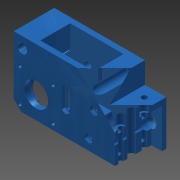
# Autodesk Inventor part: YAxisMotorBlock
Saved by Autodesk Inventor 2015 (Build 190159000, 159)
## iProperties
Created: 2014-08-06
Part Number: YAxisMotorBlock
Material: ABS Plastic
Document SubType Name: Modeling
Designer: t_clevj
Density: 1.06 g/cm^3
Appearance: Cyan
Author: t_clevj
Autodesk Inventor part; units mm, degrees
ref_plane "YZ Plane" through (0, 0, 0) normal (1, 0, 0) x (0, 1, 0)
ref_plane "XZ Plane" through (0, 0, 0) normal (0, 1, 0) x (-1, 0, 0)
ref_plane "XY Plane" through (0, 0, 0) normal (0, 0, 1) x (1, 0, 0)
sketch "Sketch1" plane through (0, 0, 0) normal (0, 1, 0) x (-1, 0, 0)
  line L0 (0, 0) -> (105, 0)
  line L1 (105, 0) -> (105, 62)
  line L2 (105, 62) -> (20, 62)
  line L3 (20, 62) -> (20, 42)
  line L4 (20, 42) -> (0, 42)
  line L5 (0, 42) -> (0, 0)
  dimension "d0" = 105
  dimension "d1" = 62
  dimension "d2" = 85
  dimension "d3" = 20
  constraints: 12 end point, 4 perpendicular, 2 horizontal
  measures "d0" distance of L0.start L0.end
  measures "d1" distance of L0.end L1.end
  measures "d2" distance of L1.end L2.end
  measures "d3" distance of L2.end L3.end
extrude "BottomFace" add sketch "Sketch1" along normal blind 5
sketch "Sketch2" plane through (0, 5, 0) normal (0, 1, 0) x (1, 0, 0)
  line L0 (0, 0) -> (-105, 0) projected
  line L1 (-105, 0) -> (-105, -62) projected
  line L2 (-93, -6.5778) -> (-93, 0)
  line L3 (-105, -62) -> (-20, -62) projected
  line L4 (-85, -62) -> (-85, -37.9706)
  arc A0 (-93, -6.5778) -> (-85, -37.9706) centre (-84, -21) ccw
  line L5 (-20, -42) -> (0, -42) projected
  line L6 (-20, -62) -> (-20, -42) projected
  line L7 (0, -42) -> (0, 0) projected
  arc A1 (-30, -46) -> (-19, -35) centre (-30, -35) ccw
  line L8 (-19, -35) -> (-19, 0)
  line L9 (-35, -46) -> (-35, -62)
  line L10 (-30, -46) -> (-35, -46)
  line L11 (-46, -10) -> (-71.0385, -10)
  line L12 (-73, -8.0385) -> (-73, 0)
  arc A2 (-42.5498, -2) -> (-46, -10) centre (-35, -10) ccw
  line L13 (-42.5498, -2) -> (-42.5498, 0)
  arc A3 (-71.0385, -10) -> (-73, -8.0385) centre (-84, -21) ccw
  dimension "d30" = 34
  dimension "d31" = 21
  dimension "d32" = 21
  dimension "d33" = 20
  dimension "d35" = 12
  dimension "d38" = 22
  dimension "d39" = 27
  dimension "d40" = 30
  dimension "d41" = 15
  dimension "d44" = 20
  dimension "d45" = 22
  dimension "d46" = 10
  dimension "d47" = 35
  dimension "d48" = 2
  dimension "d51" = 17
  dimension "d52" = 10
  constraints: 16 end point, 8 point on circle, 6 perpendicular, 6 point on line, 4 centre point, 2 tangent, 1 coincident, 1 horizontal, 1 vertical
  measures "d30" diameter of A0
  measures "d31" distance from line of L1 A0.centre
  measures "d32" distance from line of L0 A0.centre
  measures "d33" distance between parallel lines of L1 L4
  measures "d35" distance from line of L0.end L2
  measures "d38" diameter of A1
  measures "d39" distance from line of L3 A1.centre
  measures "d40" distance from line of L7 A1.centre
  measures "d41" distance between parallel lines of L6 L9
  measures "d44" distance between parallel lines of L2 L12
  measures "d45" diameter of A2
  measures "d46" distance from line of L0 A2.centre
  measures "d47" distance from line of L7 A2.centre
  measures "d48" distance of L13.start L13.end
  measures "d51" radius of A3
  measures "d52" distance between parallel lines of L0 L11
extrude "Extrusion9" add sketch "Sketch2" along normal blind 28 contours L7 L5 L6 L3 L9 L10 A1 L8 L0 | L13 A2 L11 A3 L12 L0 | L2 A0 L4 L3 L1 L0
sketch "Sketch8" plane through (0, 5, 0) normal (0, 1, 0) x (1, 0, 0)
  arc A0 (-93, -6.5778) -> (-85, -37.9706) centre (-84, -21) ccw projected
  circle A1 centre (-84, -21) radius 11.25
  line L0 (-105, 0) -> (-105, -62) projected
  line L1 (-42.5498, 0) -> (-73, 0) projected
  point P0 (0, 0)
  dimension "d53" = 22.5
  constraints: 1 centre point, 1 coincident
  measures "d53" diameter of A1
extrude "Extrusion10" cut sketch "Sketch8" against normal up to next
sketch "Sketch9" plane through (0, 33, 0) normal (0, 1, 0) x (1, 0, 0)
  line L0 (-20, -42) -> (0, -42) projected
  line L1 (0, -42) -> (0, 0) projected
  line L2 (0, 0) -> (-105, 0) projected
  line L3 (-10, 0) -> (-10, -37)
  line L4 (-10, -37) -> (0, -37)
  dimension "d62" = 5
  dimension "d63" = 10
  constraints: 4 end point, 2 point on line, 1 perpendicular, 1 vertical
  measures "d62" distance between parallel lines of L0 L4
  measures "d63" distance between parallel lines of L1 L3
extrude "Extrusion11" cut sketch "Sketch9" against normal up to next
sketch "Sketch10" plane through (0, 33, 0) normal (0, 1, 0) x (1, 0, 0)
  line L0 (0, -37) -> (-10, -37) projected
  line L1 (-10, -37) -> (-10, 0) projected
  line L2 (-20, -62) -> (-20, -42) projected
  line L3 (-20, -42) -> (0, -42) projected
  line L4 (0, -42) -> (0, -37) projected
  line L5 (-105, 0) -> (-105, -62) projected
  line L6 (-105, -62) -> (-85, -62) projected
  line L7 (-85, -62) -> (-85, -37.9706) projected
  arc A0 (-93, -6.5778) -> (-85, -37.9706) centre (-84, -21) ccw projected
  line L8 (-93, -6.5778) -> (-93, 0) projected
  line L9 (-93, 0) -> (-105, 0) projected
  line L10 (-71.0385, -10) -> (-46, -10) projected
  arc A1 (-42.5498, -2) -> (-46, -10) centre (-35, -10) ccw projected
  line L11 (-42.5498, -2) -> (-42.5498, 0) projected
  line L12 (-42.5498, 0) -> (-73, 0) projected
  line L13 (-73, 0) -> (-73, -8.0385) projected
  arc A2 (-71.0385, -10) -> (-73, -8.0385) centre (-84, -21) ccw projected
  line L14 (-20, -62) -> (-105, -62)
  line L15 (-105, -62) -> (-105, 0)
  line L16 (-105, 0) -> (-10, 0)
  point P0 (0, 0)
  constraints: 6 end point, 1 collinear, 1 horizontal, 1 perpendicular
extrude "Extrusion12" add sketch "Sketch10" along normal blind 5
sketch "Sketch11" plane through (0, 5, 0) normal (0, 1, 0) x (1, 0, 0)
  arc A0 (-30, -46) -> (-19, -35) centre (-30, -35) ccw projected
  arc A1 (-42.5498, -2) -> (-46, -10) centre (-35, -10) ccw projected
  circle A2 centre (-35, -10) radius 2.25
  circle A3 centre (-30, -35) radius 2.25
  point P0 (0, 0)
  dimension "d68" = 4.5
  dimension "d69" = 4.5
  constraints: 2 centre point, 2 coincident
  measures "d68" diameter of A2
  measures "d69" diameter of A3
extrude "Extrusion13" cut sketch "Sketch11" along normal blind 39.5 and the other way blind 5
sketch "Sketch13" plane through (0, 38, 0) normal (0, 1, 0) x (1, 0, 0)
  circle A0 centre (-99.5, -5.5) radius 1.75
  circle A1 centre (-68.5, -5.5) radius 1.75
  circle A2 centre (-68.5, -36.5) radius 1.75
  circle A3 centre (-99.5, -36.5) radius 1.75
  circle A4 centre (-84, -21) radius 11.25 projected
  point P0 (0, 0)
  dimension "d78" = 3.5
  dimension "d79" = 31
  dimension "d80" = 31
  dimension "d81" = 15.5
  dimension "d82" = 15.5
  constraints: 4 centre point, 3 equal radius, 2 horizontal alignment, 2 vertical alignment
  measures "d78" diameter of A0
  measures "d79" distance of A0.centre A1.centre
  measures "d80" distance of A2.centre A1.centre
  measures "d81" horizontal distance of A4.centre A2.centre
  measures "d82" horizontal distance of A4.centre A1.centre
hole "Hole1" at (-68.5, 38, 36.5) at (-68.5, 38, 5.5) at (-99.5, 38, 5.5) at (-99.5, 38, 36.5) direction (0, -1, 0) diameter 3.5 end up to face face through (-68.3369, 0, 51.8396) facing (0, -1, 0) counterbore diameter 6 counterbore depth 34
sketch "Sketch14" plane through (0, 0, 0) normal (0, -1, 0) x (1, 0, 0)
  line L0 (-20, 62) -> (-20, 42) projected
  line L1 (-105, 62) -> (-20, 62) projected
  line L2 (-105, 0) -> (-105, 62) projected
  circle A0 centre (-97, 52) radius 2.5
  circle A1 centre (-28, 52) radius 2.5
  point P0 (0, 0)
  dimension "d90" = 5
  dimension "d91" = 5
  dimension "d92" = 10
  dimension "d93" = 8
  dimension "d94" = 8
  constraints: 2 centre point, 1 horizontal alignment
  measures "d90" diameter of A0
  measures "d91" diameter of A1
  measures "d92" distance from line of L1 A1.centre
  measures "d93" distance from line of L2 A0.centre
  measures "d94" distance from line of L0 A1.centre
hole "Hole2" at (-28, 0, 52) at (-97, 0, 52) direction (0, 1, 0) diameter 5.5 end up to face face through (-64.3795, 38, 54.4927) facing (0, 1, 0) counterbore diameter 9 counterbore depth 33
fillet "Fillet1" radius 5 2 edges at (-35, 19, 46) (-85, 19, 37.9706)
sketch "Sketch15" plane through (0, 38, 0) normal (0, 1, 0) x (1, 0, 0)
  line L0 (-10, 0) -> (-105, 0) projected
  line L1 (-105, 0) -> (-105, -62) projected
  line L2 (-56.5, -38) -> (-56.5, -23) construction
  line L3 (-54.25, -38) -> (-54.25, -23)
  line L4 (-58.75, -23) -> (-58.75, -38)
  arc A0 (-58.75, -38) -> (-54.25, -38) centre (-56.5, -38) ccw
  arc A1 (-54.25, -23) -> (-58.75, -23) centre (-56.5, -23) ccw
  circle A2 centre (-56.5, -38) radius 3.5 construction
  point P0 (0, 0)
  point P1 (-56.5, -30.5)
  dimension "d103" = 7.5
  dimension "d104" = 4.5
  dimension "d105" = 48.5
  dimension "d106" = 23
  dimension "d118" = 7
  constraints: 8 end point, 4 point on circle, 4 tangent, 3 centre point, 1 coincident, 1 midpoint, 1 parallel, 1 vertical
  measures "d103" distance of point (-56.5, -30.5) L2.end
  measures "d104" diameter of A1
  measures "d105" distance between parallel lines of L1 L2
  measures "d106" distance from line of L0 L2.end
  measures "d118" diameter of A2
extrude "Extrusion15" cut sketch "Sketch15" against normal up to surface (38 mm away)
sketch "Sketch16" plane through (0, 0, 0) normal (0, -1, 0) x (1, 0, 0)
  line L0 (-54.25, 38) -> (-54.25, 23) projected
  arc A0 (-58.75, 23) -> (-54.25, 23) centre (-56.5, 23) ccw projected
  line L1 (-58.75, 23) -> (-58.75, 38) projected
  arc A1 (-54.25, 38) -> (-58.75, 38) centre (-56.5, 38) ccw projected
  line L2 (-56.5, 42.0415) -> (-53, 40.0207)
  line L3 (-53, 40.0207) -> (-53, 35.9793)
  line L4 (-53, 35.9793) -> (-56.5, 33.9585)
  line L5 (-56.5, 33.9585) -> (-60, 35.9793)
  line L6 (-60, 35.9793) -> (-60, 40.0207)
  line L7 (-60, 40.0207) -> (-56.5, 42.0415)
  line L8 (-56.5, 18.9585) -> (-60, 20.9793)
  line L9 (-60, 20.9793) -> (-60, 25.0207)
  line L10 (-60, 25.0207) -> (-56.5, 27.0415)
  line L11 (-56.5, 27.0415) -> (-53, 25.0207)
  line L12 (-53, 25.0207) -> (-53, 20.9793)
  line L13 (-53, 20.9793) -> (-56.5, 18.9585)
  line L14 (-60, 35.9793) -> (-60, 25.0207)
  line L15 (-53, 35.9793) -> (-53, 25.0207)
  point P0 (0, 0)
  dimension "d109" = 7
  constraints: 28 end point, 3 vertical, 2 coincident, 1 collinear, 1 vertical alignment, 26 other
  measures "d109" distance between parallel lines of L9 L12
extrude "Extrusion16" cut sketch "Sketch16" against normal blind 3.2
sketch "Sketch17" plane through (0, 0, 0) normal (0, -1, 0) x (1, 0, 0)
  circle A0 centre (-35, 10) radius 2.25 projected
  circle A1 centre (-30, 35) radius 2.25 projected
  line L0 (-35, 5.9585) -> (-38.5, 7.9793)
  line L1 (-38.5, 7.9793) -> (-38.5, 12.0207)
  line L2 (-38.5, 12.0207) -> (-35, 14.0415)
  line L3 (-35, 14.0415) -> (-31.5, 12.0207)
  line L4 (-31.5, 12.0207) -> (-31.5, 7.9793)
  line L5 (-31.5, 7.9793) -> (-35, 5.9585)
  line L6 (-30, 30.9585) -> (-33.5, 32.9793)
  line L7 (-33.5, 32.9793) -> (-33.5, 37.0207)
  line L8 (-33.5, 37.0207) -> (-30, 39.0415)
  line L9 (-30, 39.0415) -> (-26.5, 37.0207)
  line L10 (-26.5, 37.0207) -> (-26.5, 32.9793)
  line L11 (-26.5, 32.9793) -> (-30, 30.9585)
  point P0 (0, 0)
  dimension "d112" = 7
  constraints: 24 end point, 2 coincident, 2 vertical, 1 parallel, 26 other
  measures "d112" distance between parallel lines of L10 L7
extrude "Extrusion17" cut sketch "Sketch17" against normal blind 3.2
sketch "Sketch18" plane through (-10, 0, 0) normal (0, 0, -1) x (-1, 0, 0)
  line L0 (0, 38) -> (0, 0) projected
  circle A0 centre (0, 15.5) radius 4
  line L1 (0, 38) -> (95, 38) projected
  line L2 (0, 38) -> (0, 0) projected
  point P0 (-10, 0)
  dimension "d115" = 8
  dimension "d192" = 22.5
  constraints: 1 centre point, 1 point on line
  measures "d115" diameter of A0
  measures "d192" distance from line of L1 A0.centre
extrude "Extrusion18" cut sketch "Sketch18" against normal up to surface (37 mm away)
sketch "Sketch21" plane through (0, 0, 37) normal (0, 0, -1) x (-1, 0, 0)
  line L0 (0, 38) -> (10, 38) projected
  line L1 (10, 0) -> (0, 0) projected
  line L2 (10, 11.5) -> (10, 0) projected
  circle A0 centre (10, 30) radius 4.25
  circle A1 centre (10, 8) radius 4.25
  line L3 (10, 38) -> (10, 19.5) projected
  dimension "d125" = 8.5
  dimension "d126" = 8.5
  dimension "d127" = 8
  dimension "d128" = 8
  constraints: 2 centre point, 2 point on line
  measures "d125" diameter of A0
  measures "d126" diameter of A1
  measures "d127" distance from line of L0 A0.centre
  measures "d128" distance from line of L1 A1.centre
extrude "Extrusion21" [suppressed]
sketch "Sketch22" plane through (-10, 30, 37) normal (0, 0, -1) x (-1, 0, 0)
  circle A0 centre (0, 0) radius 4.25 projected
  circle A1 centre (0, -22) radius 4.25 projected
  circle A2 centre (0, -22) radius 2.5
  circle A3 centre (0, 0) radius 2.5
  point P0 (-10, -30)
  dimension "d133" = 5
  dimension "d134" = 5
  constraints: 2 centre point, 2 coincident
  measures "d133" diameter of A2
  measures "d134" diameter of A3
extrude "Extrusion22" [suppressed]
sketch "Sketch23" plane through (0, 38, 0) normal (0, 1, 0) x (1, 0, 0)
  line L0 (-54.25, -23) -> (-54.25, -38) projected
  arc A0 (-58.75, -38) -> (-54.25, -38) centre (-56.5, -38) ccw projected
  line L1 (-58.75, -38) -> (-58.75, -23) projected
  arc A1 (-54.25, -23) -> (-58.75, -23) centre (-56.5, -23) ccw projected
  line L2 (-56.5, -38) -> (-56.5, -23) construction
  line L3 (-53, -38) -> (-53, -23)
  line L4 (-60, -23) -> (-60, -38)
  arc A2 (-60, -38) -> (-53, -38) centre (-56.5, -38) ccw
  arc A3 (-53, -23) -> (-60, -23) centre (-56.5, -23) ccw
  point P0 (0, 0)
  point P1 (-56.5, -30.5)
  dimension "d137" = 7
  constraints: 8 end point, 4 point on circle, 4 tangent, 2 centre point, 1 midpoint, 1 parallel, 1 vertical
  measures "d137" diameter of A3
extrude "Extrusion23" cut sketch "Sketch23" against normal blind 4
sketch "Sketch24" plane through (-10, 38, 37) normal (1, 0, 0) x (0, 0, -1)
  line L0 (37, 0) -> (37, -18.5) projected
  line L1 (0, 0) -> (0, -18.5) projected
  line L2 (37, -38) -> (0, -38) projected
  line L3 (37, -26.5) -> (37, -38) projected
  line L4 (37, -26.5) -> (0, -26.5) projected
  circle A0 centre (31, -10.5) radius 2
  circle A1 centre (31, -32.5) radius 2
  line L5 (0, -26.5) -> (0, -38) projected
  line L6 (0, -18.5) -> (37, -18.5) projected
  line L7 (37, 0) -> (37, -18.5) projected
  line L8 (0, 0) -> (37, 0) projected
  dimension "d140" = 4
  dimension "d141" = 4
  dimension "d144" = 6
  dimension "d210" = 5.5
  dimension "d212" = 27.5
  constraints: 2 centre point, 1 vertical alignment
  measures "d140" diameter of A0
  measures "d141" diameter of A1
  measures "d144" distance from line of L0 A0.centre
  measures "d210" distance from line of L2 A1.centre
  measures "d212" distance from line of L2 A0.centre
extrude "Extrusion24" cut sketch "Sketch24" against normal up to surface (9 mm away) contours A0 | A1
sketch "Sketch25" plane through (-10, 38, 37) normal (1, 0, 0) x (0, 0, -1)
  line L0 (37, 0) -> (37, -18.5) projected
  line L1 (0, 0) -> (37, 0) projected
  line L2 (0, 0) -> (0, -18.5) projected
  line L3 (0, -4) -> (37, -4)
  dimension "d147" = 4
  constraints: 2 end point, 2 point on line, 1 perpendicular
  measures "d147" distance between parallel lines of L1 L3
extrude "Extrusion25" add sketch "Sketch25" along normal blind 10
sketch "Sketch26" plane through (-10, 34, 0) normal (0, -1, 0) x (1, 0, 0)
  line L0 (0, 0) -> (10, 0) projected
  line L1 (10, 37) -> (10, 0) projected
  circle A0 centre (0, 18.5) radius 2.5
  dimension "d150" = 5
  dimension "d151" = 10
  dimension "d152" = 18.5
  constraints: 1 centre point
  measures "d150" diameter of A0
  measures "d151" distance from line of L1 A0.centre
  measures "d152" distance from line of L0 A0.centre
extrude "Extrusion26" cut sketch "Sketch26" against normal up to next
sketch "Sketch27" plane through (0, 0, 37) normal (0, 0, -1) x (-1, 0, 0)
  line L0 (0, 0) -> (0, 34) projected
  circle A0 centre (10, 27.5) radius 2.5
  circle A1 centre (10, 5.5) radius 2.5
  line L1 (10, 0) -> (0, 0) projected
  dimension "d155" = 5
  dimension "d156" = 5
  dimension "d157" = 10
  dimension "d207" = 5.5
  dimension "d208" = 27.5
  constraints: 2 centre point, 1 vertical alignment
  measures "d155" diameter of A0
  measures "d156" diameter of A1
  measures "d157" distance from line of L0 A0.centre
  measures "d207" distance from line of L1 A1.centre
  measures "d208" distance from line of L1 A0.centre
extrude "Extrusion27" cut sketch "Sketch27" against normal up to next
sketch "Sketch28" plane through (-10, 0, 0) normal (0, 0, -1) x (-1, 0, 0)
  circle A0 centre (0, 27.5) radius 2.5 projected
  arc A1 (0, 25) -> (0, 30) centre (0, 27.5) ccw projected
  arc A2 (0, 30) -> (0, 25) centre (0, 27.5) ccw projected
  circle A3 centre (0, 5.5) radius 2.5 projected
  arc A4 (0, 3) -> (0, 8) centre (0, 5.5) ccw projected
  arc A5 (0, 8) -> (0, 3) centre (0, 5.5) ccw projected
  point P0 (-10, 0)
extrude "Extrusion28" cut sketch "Sketch28" against normal blind 37
sketch "Sketch29" plane through (0, 0, 37) normal (0, 0, -1) x (-1, 0, 0)
  circle A0 centre (10, 27.5) radius 2.5 projected
  circle A1 centre (10, 27.5) radius 4.25
  circle A2 centre (10, 5.5) radius 2.5 projected
  circle A3 centre (10, 5.5) radius 4.25
  dimension "d165" = 8.5
  dimension "d166" = 8.5
  constraints: 2 centre point, 2 coincident
  measures "d165" diameter of A1
  measures "d166" diameter of A3
extrude "Extrusion29" cut sketch "Sketch29" along normal blind 9 contours A0 | A1 | A2 | A3
sketch "Sketch31" plane through (0, 38, 0) normal (0, 1, 0) x (1, 0, 0)
  circle A0 centre (-35, -10) radius 2.25 projected
  circle A1 centre (-30, -35) radius 2.25 projected
  circle A2 centre (-35, -10) radius 3.5
  circle A3 centre (-30, -35) radius 3.5
  dimension "d177" = 7
  dimension "d178" = 7
  constraints: 2 centre point, 2 coincident
  measures "d177" diameter of A2
  measures "d178" diameter of A3
extrude "Extrusion31" cut sketch "Sketch31" against normal blind 4
sketch "Sketch32" plane through (-10, 34, 16) normal (1, 0, 0) x (0, 0, -1)
  line L0 (16, 0) -> (0, 0) projected
  line L1 (0, 0) -> (0, 4) projected
  line L2 (-5, 4) -> (0, 4) projected
  line L3 (-5, 0) -> (0, 0) projected
  line L4 (0, 0) -> (-5, 0) projected
  line L5 (0, 2.5) -> (2.5, 0)
  line L6 (0, 2.5) -> (0, 0)
  line L7 (0, 0) -> (2.5, 0)
  line L8 (-2.5, 4) -> (-2.5, 0)
  point P0 (16, -34)
  dimension "d181" = 2.5
  dimension "d182" = 45
  constraints: 8 end point, 2 midpoint, 2 point on line, 1 collinear, 1 perpendicular
  measures "d181" distance of L0.end L5.end
  measures "d182" angle of L0 L5
revolve "Revolution1" cut sketch "Sketch32" angle 360 about axis through (-10, 38, 18.5) along (0, -1, 0) contours L0 L1 L5
sketch "Sketch33" plane through (-10, 34, 0) normal (0, -1, 0) x (1, 0, 0)
  arc A0 (0, 13.5) -> (0, 23.5) centre (0, 18.5) ccw projected
  circle A1 centre (0, 18.5) radius 5
  point P0 (2, 13.9174)
  point P1 (2, 23.0826)
  constraints: 1 centre point, 1 coincident, 1 concentric
extrude "Extrusion32" cut sketch "Sketch33" along normal blind 8
sketch "Sketch34" plane through (-10, 34, 0) normal (0, -1, 0) x (1, 0, 0)
  arc A0 (0, 13.5) -> (0, 23.5) centre (0, 18.5) ccw projected
  circle A1 centre (0, 18.5) radius 1.8
  point P0 (2, 13.9174)
  point P1 (2, 23.0826)
  dimension "d186" = 3.6
  constraints: 1 centre point, 1 coincident
  measures "d186" diameter of A1
extrude "Extrusion33" cut sketch "Sketch34" along normal up to surface (34 mm away)
sketch "Sketch37" plane through (-10, 19.5, 37) normal (1, 0, 0) x (0, 0, -1)
  circle A0 centre (13, 8) radius 2
  circle A1 centre (13, -14) radius 2
  line L0 (37, -8) -> (37, -19.5) projected
  line L1 (16.7, -19.5) -> (0, -19.5) projected
  dimension "d200" = 4
  dimension "d201" = 4
  dimension "d203" = 24
  dimension "d204" = 5.5
  dimension "d209" = 27.5
  constraints: 2 centre point, 1 vertical alignment
  measures "d200" diameter of A0
  measures "d201" diameter of A1
  measures "d203" distance from line of L0 A1.centre
  measures "d204" distance from line of L1 A1.centre
  measures "d209" distance from line of L1 A0.centre
extrude "Extrusion36" cut sketch "Sketch37" against normal up to surface (9 mm away)
sketch "Sketch38" plane through (-19, 5, 35) normal (-1, 0, 0) x (0, 0, 1)
  circle A0 centre (-29, 22.5) radius 2 projected
  arc A1 (-9.0635, 0) -> (-12.9365, 0) centre (-11, 0.5) ccw projected
  arc A2 (-27.0635, 0) -> (-30.9365, 0) centre (-29, 0.5) ccw projected
  circle A3 centre (-11, 22.5) radius 2 projected
  line L0 (-24.9585, 22.5) -> (-26.9793, 19)
  line L1 (-26.9793, 19) -> (-31.0207, 19)
  line L2 (-31.0207, 19) -> (-33.0415, 22.5)
  line L3 (-33.0415, 22.5) -> (-31.0207, 26)
  line L4 (-31.0207, 26) -> (-26.9793, 26)
  line L5 (-26.9793, 26) -> (-24.9585, 22.5)
  line L6 (-24.9585, 0.5) -> (-26.9793, -3)
  line L7 (-26.9793, -3) -> (-31.0207, -3)
  line L8 (-31.0207, -3) -> (-33.0415, 0.5)
  line L9 (-33.0415, 0.5) -> (-31.0207, 4)
  line L10 (-31.0207, 4) -> (-26.9793, 4)
  line L11 (-26.9793, 4) -> (-24.9585, 0.5)
  line L12 (-6.9585, 0.5) -> (-8.9793, -3)
  line L13 (-8.9793, -3) -> (-13.0207, -3)
  line L14 (-13.0207, -3) -> (-15.0415, 0.5)
  line L15 (-15.0415, 0.5) -> (-13.0207, 4)
  line L16 (-13.0207, 4) -> (-8.9793, 4)
  line L17 (-8.9793, 4) -> (-6.9585, 0.5)
  line L18 (-6.9585, 22.5) -> (-8.9793, 19)
  line L19 (-8.9793, 19) -> (-13.0207, 19)
  line L20 (-13.0207, 19) -> (-15.0415, 22.5)
  line L21 (-15.0415, 22.5) -> (-13.0207, 26)
  line L22 (-13.0207, 26) -> (-8.9793, 26)
  line L23 (-8.9793, 26) -> (-6.9585, 22.5)
  point P0 (-35, -5)
  dimension "d213" = 7
  dimension "d214" = 7
  dimension "d215" = 7
  dimension "d216" = 7
  constraints: 48 end point, 4 coincident, 4 horizontal, 52 other
  measures "d213" distance between parallel lines of L19 L22
  measures "d214" distance between parallel lines of L1 L4
  measures "d215" distance between parallel lines of L7 L10
  measures "d216" distance between parallel lines of L13 L16
extrude "Extrusion37" cut sketch "Sketch38" against normal blind 3.2 and the other way blind 4
body "Solid1"
